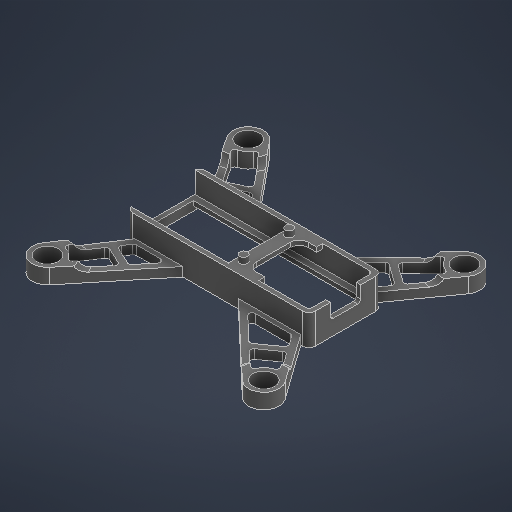
# Autodesk Inventor part: P_DroneCase
Saved by Autodesk Inventor 2026 (Build 300175000, 175)
## iProperties
Created: 2025-08-01
Part Number: P_DroneCase
Material: Generisch
Document SubType Name: Modeling
Designer: FAL
Density: 1 g/cm^3
Appearance: Vorgabe
Author: FAL
Autodesk Inventor part; units mm, degrees
ref_plane "YZ Plane" through (0, 0, 0) normal (1, 0, 0) x (0, 1, 0)
ref_plane "XZ Plane" through (0, 0, 0) normal (0, 1, 0) x (-1, 0, 0)
ref_plane "XY Plane" through (0, 0, 0) normal (0, 0, 1) x (1, 0, 0)
sketch "Skizze1" plane through (0, 0, 0) normal (0, 0, 1) x (1, 0, 0)
  line L0 (-30, 0) -> (30, 0)
  line L1 (30, 0) -> (30, -12)
  line L2 (30, -12) -> (-30, -12)
  line L3 (-30, -12) -> (-30, 0)
  line L4 (0, 0) -> (0, -12) construction
  dimension "d0" = 60
  dimension "d1" = 12
  constraints: 10 end point, 3 midpoint, 2 parallel, 1 horizontal, 1 perpendicular, 1 point on line
  measures "d0" distance of L1.end L2.end
  measures "d1" distance between parallel lines of L0 L2
extrude "Extrusion1" add sketch "Skizze1" along normal blind 10
fillet "Rundung1" radius 2 2 edges at (-30, -12, 5) (30, -12, 5)
sketch "Skizze2" plane through (0, 0, 0) normal (0, 0, 1) x (1, 0, 0)
  line L0 (-31.1249, -36.1597) -> (-1.6411, 0)
  line L1 (-19.3399, 0) -> (-39.1812, -30.2582)
  arc A0 (-39.1812, -30.2582) -> (-31.1249, -36.1597) centre (-35, -33) ccw
  line L2 (30, 0) -> (-30, 0) projected
  line L3 (18.704, 0) -> (40.2164, -30.0922)
  arc A1 (32.7035, -36.6234) -> (40.2164, -30.0922) centre (36.1489, -33) ccw
  line L4 (-1.6411, 0) -> (18.704, 0)
  line L5 (32.7035, -36.6234) -> (-5.8126, 0)
  line L6 (-19.3399, 0) -> (-1.6411, 0)
  line L7 (-5.8126, 0) -> (18.704, 0)
  point P0 (0, 0)
  point P1 (0, 0)
  point P2 (0, 0)
  point P3 (0, 0)
  dimension "d10" = 35
  dimension "d12" = 5
  dimension "d19" = 5
  dimension "d38" = 33
  dimension "d39" = 33
  constraints: 15 end point, 4 point on circle, 4 tangent, 2 centre point, 1 collinear, 1 horizontal, 1 point on line, 6 other
  measures "d10" horizontal distance of point (0, 0) A0.centre
  measures "d12" radius of A0
  measures "d19" radius of A1
extrude "Extrusion2" add sketch "Skizze2" along normal blind 3
sketch "Skizze12" plane through (0, 0, 3) normal (0, 0, 1) x (1, 0, 0)
  line L0 (-27.2087, -12) -> (-11.4256, -12) projected
  line L1 (-27.2087, -12) -> (-39.1812, -30.2582) projected
  arc A0 (-39.1812, -30.2582) -> (-31.1249, -36.1597) centre (-35, -33) ccw projected
  line L2 (-31.1249, -36.1597) -> (-11.4256, -12) projected
  line L3 (6.8076, -12) -> (27.2826, -12) projected
  line L4 (6.8076, -12) -> (32.7035, -36.6234) projected
  arc A1 (32.7035, -36.6234) -> (40.2164, -30.0922) centre (36.1489, -33) ccw projected
  line L5 (40.2164, -30.0922) -> (27.2826, -12) projected
  circle A2 centre (-35, -33) radius 7.5
  circle A3 centre (36.1489, -33) radius 7.5
  point P0 (0, 0)
  point P1 (36.9654, -25.5446)
  point P2 (28.6524, -32.7714)
  point P3 (-27.5923, -31.8272)
  point P4 (-36.1158, -25.5835)
  dimension "d73" = 15
  constraints: 2 centre point, 2 coincident, 1 equal radius
  measures "d73" diameter of A3
extrude "Extrusion10" add sketch "Skizze12" along normal blind 2 contours A2 L2 A0 L1 | A3 L5 A1 L4 picked at (-33.4092, -31.2997) picked at (34.9492, -31.1721)
fillet "Rundung6" radius 3 2 edges at (-30.568, -26.9496, 3) (31.2283, -27.3398, 3)
sketch "Skizze3" plane through (0, 0, 0) normal (0, 0, 1) x (1, 0, 0)
  arc A0 (-39.1812, -30.2582) -> (-31.1249, -36.1597) centre (-35, -33) ccw projected
  circle A1 centre (-35, -33) radius 3.6
  arc A2 (32.7035, -36.6234) -> (40.2164, -30.0922) centre (36.1489, -33) ccw projected
  circle A3 centre (36.1489, -33) radius 3.6
  point P0 (0, 0)
  dimension "d16" = 7.2
  constraints: 2 centre point, 2 coincident, 1 equal radius
  measures "d16" diameter of A1
extrude "Extrusion3" cut sketch "Skizze3" along normal blind 5
sketch "Skizze4" plane through (0, 0, 3) normal (0, 0, 1) x (1, 0, 0)
  line L0 (-25.8007, -13.5) -> (-15.2293, -13.5)
  line L1 (-15.2293, -13.5) -> (-30.1472, -31.7957)
  line L2 (-35.3153, -28.01) -> (-25.8007, -13.5)
  line L3 (11.2875, -13.5) -> (25.8964, -13.5)
  line L4 (25.8964, -13.5) -> (36.2631, -28.0013)
  line L5 (31.1829, -32.4178) -> (11.2875, -13.5)
  circle A0 centre (36.1489, -33) radius 3.6 projected
  arc A1 (36.2631, -28.0013) -> (31.1829, -32.4178) centre (36.1489, -33) ccw
  arc A2 (-39.1812, -30.2582) -> (-31.1249, -36.1597) centre (-35, -33) ccw projected
  arc A3 (-30.1472, -31.7957) -> (-35.3153, -28.01) centre (-35, -33) ccw
  line L6 (40.2164, -30.0922) -> (27.2826, -12) projected
  line L7 (-28, -12) -> (28, -12) projected
  line L8 (-31.1249, -36.1597) -> (-11.4256, -12) projected
  line L9 (-27.2087, -12) -> (-39.1812, -30.2582) projected
  line L10 (6.8076, -12) -> (32.7035, -36.6234) projected
  line L11 (29.9581, -19.1816) -> (22.7111, -24.3623)
  line L12 (28.7949, -17.5545) -> (21.2352, -22.9589)
  line L13 (-20.8604, -20.4061) -> (-28.1066, -17.0166)
  line L14 (-22.1636, -22.0045) -> (-29.2146, -18.7064)
  point P0 (0, 0)
  point P1 (22.5, -5.3099)
  point P2 (-22.5, -4.8192)
  point P3 (-25.7908, 0)
  point P4 (28.6377, -13.8956)
  point P5 (-28.4816, -13.9412)
  dimension "d23" = 5
  dimension "d24" = 5
  dimension "d25" = 1.5
  dimension "d26" = 1.5
  dimension "d28" = 2
  dimension "d29" = 2
  dimension "d30" = 2
  dimension "d40" = 2
  dimension "d71" = 2
  dimension "d72" = 2
  constraints: 20 end point, 7 parallel, 7 point on line, 4 point on circle, 2 centre point, 2 coincident, 1 horizontal, 1 midpoint, 1 perpendicular, 2 other
  measures "d23" radius of A3
  measures "d24" radius of A1
  measures "d25" distance between parallel lines of L7 L3
  measures "d26" distance between parallel lines of L7 L0
  measures "d28" distance between parallel lines of L6 L4
  measures "d29" distance between parallel lines of L8 L1
  measures "d40" distance between parallel lines of L10 L5
  measures "d71" distance between parallel lines of L12 L11
  measures "d72" distance between parallel lines of L14 L13
extrude "Extrusion4" cut sketch "Skizze4" along normal through all both and the other way through all contours L0 L1 L13 L2 | L14 L1 A3 L2 | L3 L4 L12 L5 | L11 L4 A1 L5
fillet "Rundung2" radius 1 16 edges at (-25.8007, -13.5, 1.5) (-15.2293, -13.5, 1.5) (-30.1472, -31.7957, 2.5) (-35.3153, -28.01, 2.5) (11.2875, -13.5, 1.5) (25.8964, -13.5, 1.5) (36.2631, -28.0013, 2.5) (31.1829, -32.4178, 2.5) (21.2352, -22.9589, 1.5) (28.7949, -17.5545, 1.5) (-22.1636, -22.0045, 1.5) (29.9581, -19.1816, 1.5) (22.7111, -24.3623, 1.5) (-28.1066, -17.0166, 1.5) (-20.8604, -20.4061, 1.5) (-29.2146, -18.7064, 1.5)
sketch "Skizze5" plane through (0, 0, 0) normal (0, 0, -1) x (-1, 0, 0)
  line L0 (28.5, 5) -> (-28.5, 5)
  line L1 (-28.5, 5) -> (-28.5, -10.5)
  line L2 (-28.5, -10.5) -> (28.5, -10.5)
  line L3 (28.5, -10.5) -> (28.5, 5)
  line L4 (11.4256, -12) -> (-6.8076, -12) projected
  line L5 (-30, -10) -> (-30, 0) projected
  line L6 (30, 0) -> (30, -10) projected
  line L7 (-30, 0) -> (30, 0) projected
  point P0 (0, 0)
  point P1 (-14.3473, -14)
  point P2 (-22.5, -5.3099)
  point P3 (28.5, -2.75)
  point P4 (-6.8076, -12)
  dimension "d31" = 1.5
  dimension "d32" = 1.5
  dimension "d48" = 1.5
  dimension "d49" = 5
  constraints: 8 end point, 2 parallel, 1 horizontal, 1 midpoint, 1 perpendicular, 2 other
  measures "d48" distance between parallel lines of L6 L3
  measures "d49" distance between parallel lines of L7 L0
extrude "Extrusion5" cut sketch "Skizze5" against normal blind 14.75
fillet "Rundung3" radius 1 2 edges at (-28.5, -10.5, 5) (28.5, -10.5, 5)
sketch "Skizze7" plane through (30, 0, 10) normal (1, 0, 0) x (0, 0, -1)
  line L0 (10, 0) -> (0, 0) projected
  line L1 (0, 0) -> (5, 0)
  line L2 (5, 0) -> (5, -5)
  line L3 (5, -5) -> (0, -5)
  line L4 (0, -5) -> (0, 0)
  point P0 (5, 0)
  dimension "d46" = 5
  dimension "d47" = 5
  constraints: 8 end point, 2 parallel, 1 horizontal, 1 perpendicular
  measures "d46" distance between parallel lines of L4 L2
  measures "d47" distance between parallel lines of L0 L3
extrude "Extrusion6" cut sketch "Skizze7" against normal blind 7.5
fillet "Rundung4" radius 1 1 edges at (29.25, -5, 5)
sketch "Skizze8" plane through (-30, 0, 0) normal (-1, 0, 0) x (0, 0, 1)
  line L0 (0, 0) -> (10, 0) projected
  line L1 (10, 0) -> (3, 0)
  line L2 (3, 0) -> (3, -10.5)
  line L3 (3, -10.5) -> (10, -10.5)
  line L4 (10, -10.5) -> (10, 0)
  point P0 (3, 0)
  dimension "d84" = 7
  constraints: 8 end point, 2 parallel, 1 horizontal, 1 perpendicular, 1 point on line
  measures "d84" distance between parallel lines of L4 L2
extrude "Extrusion7" cut sketch "Skizze8" against normal blind 7
sketch "Skizze9" plane through (0, 0, 10) normal (0, 0, 1) x (1, 0, 0)
  line L0 (-28, -12) -> (28, -12) projected
  line L1 (12, -12) -> (2, -12)
  line L2 (2, -12) -> (2, 0)
  line L3 (2, 0) -> (12, 0)
  line L4 (12, 0) -> (12, -12)
  line L5 (30, -10) -> (30, -5) projected
  point P0 (0, 0)
  dimension "d81" = 10
  dimension "d82" = 18
  constraints: 8 end point, 2 parallel, 2 point on line, 1 horizontal, 1 perpendicular
  measures "d81" distance between parallel lines of L2 L4
  measures "d82" distance between parallel lines of L5 L4
extrude "Extrusion8" add sketch "Skizze9" against normal blind 1.5
sketch "Skizze11" plane through (0, 0, 10) normal (0, 0, 1) x (1, 0, 0)
  circle A0 centre (4, -7.5) radius 1.3
  line L0 (12, 0) -> (2, 0) projected
  line L1 (2, 0) -> (2, -10.5) projected
  point P0 (0, 0)
  dimension "d56" = 2.6
  dimension "d74" = 7.5
  dimension "d75" = 2
  constraints: 1 centre point
  measures "d56" diameter of A0
  measures "d74" distance from line of L0 A0.centre
  measures "d75" distance from line of L1 A0.centre
extrude "Extrusion9" add sketch "Skizze11" along normal blind 2
sketch "Skizze16" plane through (0, 0, 10) normal (0, 0, 1) x (1, 0, 0)
  line L0 (12, -10.5) -> (12, 0) projected
  line L1 (12, 0) -> (6.3, 0)
  line L2 (6.3, 0) -> (6.3, -8.5)
  line L3 (6.3, -8.5) -> (12, -8.5)
  line L4 (12, -8.5) -> (12, 0)
  circle A0 centre (4, -7.5) radius 1.3 projected
  line L5 (27.5, -10.5) -> (12, -10.5) projected
  point P0 (0, 0)
  dimension "d76" = 1
  dimension "d77" = 2
  constraints: 8 end point, 2 parallel, 1 horizontal, 1 perpendicular
  measures "d76" distance edge to line of A0 L2
  measures "d77" distance between parallel lines of L5 L3
extrude "Extrusion13" cut sketch "Skizze16" against normal blind 4.75 contours L3 L2 L1 L0
fillet "Rundung8" radius 3 1 edges at (6.3, -8.5, 9.25)
sketch "Skizze13" plane through (-30, 0, 3) normal (0, 0, 1) x (1, 0, 0)
  arc A0 (0.0635, -10.5) -> (2, -12) centre (2, -10) ccw projected
  line L0 (2, -12) -> (58, -12) projected
  arc A1 (58, -12) -> (60, -10) centre (58, -10) ccw projected
  line L1 (60, -10) -> (60, -5) projected
  line L2 (60, -5) -> (60, -4) projected
  line L3 (60, 0) -> (60, -4) projected
  line L4 (0, 0) -> (1.5, 0) projected
  line L5 (0, 0) -> (60, 0)
  arc A2 (0, -10) -> (0.0635, -10.5) centre (2, -10) ccw projected
  line L6 (0, -10) -> (0, 0) projected
  point P0 (30, 0)
  constraints: 2 end point, 1 collinear
extrude "Extrusion11" add sketch "Skizze13" against normal blind 1.5
sketch "Skizze15" plane through (-30, 0, 1.5) normal (0, 0, -1) x (-1, 0, 0)
  line L0 (-1.5, 0) -> (-58.5, 0) projected
  line L1 (-1.5, 0) -> (-1.5, -9.5) projected
  line L2 (-58.5, 0) -> (-1.5, 0)
  line L3 (-1.5, 0) -> (-1.5, -8.5)
  line L4 (-1.5, -8.5) -> (-58.5, -8.5)
  line L5 (-58.5, -8.5) -> (-58.5, 0)
  line L6 (-2.5, -10.5) -> (-57.5, -10.5) projected
  dimension "d83" = 2
  constraints: 8 end point, 2 parallel, 1 horizontal, 1 perpendicular, 1 point on line
  measures "d83" distance between parallel lines of L4 L6
extrude "Extrusion12" cut sketch "Skizze15" against normal blind 4
mirror "Spiegeln1" about plane through (0, 0, 0) normal (0, 1, 0)
